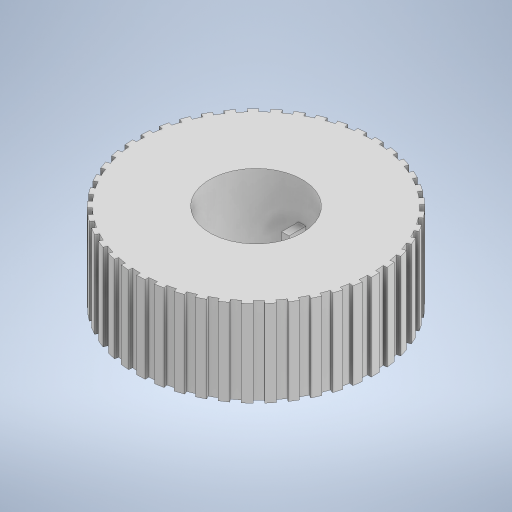
# Autodesk Inventor part: DialKnob
Saved by Autodesk Inventor 2024 (Build 280153000, 153)
## iProperties
Created: 2023-11-18
Part Number: DialKnob
Material: Generic
Document SubType Name: Modeling
Designer: gcter
Density: 1 g/cm^3
Appearance: Default
Author: gcter
Autodesk Inventor part; units mm, degrees
ref_plane "YZ Plane" through (0, 0, 0) normal (1, 0, 0) x (0, 1, 0)
ref_plane "XZ Plane" through (0, 0, 0) normal (0, 1, 0) x (-1, 0, 0)
ref_plane "XY Plane" through (0, 0, 0) normal (0, 0, 1) x (1, 0, 0)
sketch "Sketch1" plane through (0, 0, 0) normal (0, 1, 0) x (-1, 0, 0)
  arc A0 (-1.1143, -7.923) -> (-0.5589, -7.9815) centre (0, 0) ccw
  line L0 (-0.0008, -8.0004) -> (-0.0009, -8.255)
  line L1 (-0.5589, -7.9815) -> (-0.5767, -8.2348)
  circle A1 centre (0, 0) radius 8.255 construction
  line L2 (-0.0009, -8.255) -> (-0.5767, -8.2348)
  line L3 (-1.1143, -7.923) -> (-1.1497, -8.1745) construction
  line L4 (1.1126, -7.9227) -> (1.148, -8.1748)
  line L5 (1.148, -8.1748) -> (0.575, -8.235)
  line L6 (0.5573, -7.9816) -> (0.575, -8.235)
  arc A2 (-0.0008, -8.001) -> (0.5573, -7.9816) centre (0, 0) ccw
  line L7 (2.2044, -7.6907) -> (2.2746, -7.9355)
  line L8 (2.2746, -7.9355) -> (1.7155, -8.0748)
  line L9 (1.6627, -7.8263) -> (1.7155, -8.0748)
  arc A3 (1.1127, -7.9232) -> (1.6627, -7.8263) centre (0, 0) ccw
  line L10 (3.2533, -7.3091) -> (3.3568, -7.5417)
  line L11 (3.3568, -7.5417) -> (2.8226, -7.7575)
  line L12 (2.7357, -7.5188) -> (2.8226, -7.7575)
  arc A4 (2.2046, -7.6913) -> (2.7357, -7.5188) centre (0, 0) ccw
  line L13 (4.2389, -6.7852) -> (4.3738, -7.0011)
  line L14 (4.3738, -7.0011) -> (3.8747, -7.2891)
  line L15 (3.7555, -7.0649) -> (3.8747, -7.2891)
  arc A5 (3.2535, -7.3096) -> (3.7555, -7.0649) centre (0, 0) ccw
  line L16 (5.1419, -6.1292) -> (5.3056, -6.3242)
  line L17 (5.3056, -6.3242) -> (4.8515, -6.6789)
  line L18 (4.7022, -6.4734) -> (4.8515, -6.6789)
  arc A6 (4.2392, -6.7857) -> (4.7022, -6.4734) centre (0, 0) ccw
  line L19 (5.9449, -5.3539) -> (6.1341, -5.5243)
  line L20 (6.1341, -5.5243) -> (5.7338, -5.9387)
  line L21 (5.5574, -5.756) -> (5.7338, -5.9387)
  arc A7 (5.1423, -6.1297) -> (5.5574, -5.756) centre (0, 0) ccw
  line L22 (6.6322, -4.4745) -> (6.8432, -4.6168)
  line L23 (6.8432, -4.6168) -> (6.5045, -5.083)
  line L24 (6.3044, -4.9266) -> (6.5045, -5.083)
  arc A8 (5.9453, -5.3543) -> (6.3044, -4.9266) centre (0, 0) ccw
  line L25 (7.1904, -3.5079) -> (7.4192, -3.6195)
  line L26 (7.4192, -3.6195) -> (7.1486, -4.1282)
  line L27 (6.9287, -4.0012) -> (7.1486, -4.1282)
  arc A9 (6.6327, -4.4748) -> (6.9287, -4.0012) centre (0, 0) ccw
  line L28 (7.6086, -2.4731) -> (7.8507, -2.5517)
  line L29 (7.8507, -2.5517) -> (7.6536, -3.0932)
  line L30 (7.4181, -2.998) -> (7.6536, -3.0932)
  arc A10 (7.1909, -3.5082) -> (7.4181, -2.998) centre (0, 0) ccw
  line L31 (7.8787, -1.3901) -> (8.1294, -1.4343)
  line L32 (8.1294, -1.4343) -> (8.0096, -1.9979)
  line L33 (7.7631, -1.9364) -> (8.0096, -1.9979)
  arc A11 (7.6091, -2.4732) -> (7.7631, -1.9364) centre (0, 0) ccw
  line L34 (7.9955, -0.28) -> (8.2499, -0.2889)
  line L35 (8.2499, -0.2889) -> (8.2097, -0.8637)
  line L36 (7.9571, -0.8372) -> (8.2097, -0.8637)
  arc A12 (7.8793, -1.3902) -> (7.9571, -0.8372) centre (0, 0) ccw
  line L37 (7.9567, 0.8354) -> (8.2099, 0.862)
  line L38 (8.2099, 0.862) -> (8.25, 0.2872)
  line L39 (7.9962, 0.2784) -> (8.25, 0.2872)
  arc A13 (7.9961, -0.2801) -> (7.9962, 0.2784) centre (0, 0) ccw
  line L40 (7.763, 1.9347) -> (8.01, 1.9962)
  line L41 (8.01, 1.9962) -> (8.1297, 1.4326)
  line L42 (7.8796, 1.3885) -> (8.1297, 1.4326)
  arc A14 (7.9573, 0.8355) -> (7.8796, 1.3885) centre (0, 0) ccw
  line L43 (7.4182, 2.9962) -> (7.6542, 3.0916)
  line L44 (7.6542, 3.0916) -> (7.8512, 2.5501)
  line L45 (7.6097, 2.4717) -> (7.8512, 2.5501)
  arc A15 (7.7635, 1.9348) -> (7.6097, 2.4717) centre (0, 0) ccw
  line L46 (6.929, 3.9995) -> (7.1495, 4.1268)
  line L47 (7.1495, 4.1268) -> (7.4199, 3.618)
  line L48 (7.1916, 3.5067) -> (7.4199, 3.618)
  arc A16 (7.4187, 2.9965) -> (7.1916, 3.5067) centre (0, 0) ccw
  line L49 (6.3049, 4.9249) -> (6.5056, 5.0816)
  line L50 (6.5056, 5.0816) -> (6.8442, 4.6154)
  line L51 (6.6336, 4.4734) -> (6.8442, 4.6154)
  arc A17 (6.9295, 3.9998) -> (6.6336, 4.4734) centre (0, 0) ccw
  line L52 (5.5582, 5.7545) -> (5.735, 5.9376)
  line L53 (5.735, 5.9376) -> (6.1352, 5.523)
  line L54 (5.9465, 5.3531) -> (6.1352, 5.523)
  arc A18 (6.3054, 4.9253) -> (5.9465, 5.3531) centre (0, 0) ccw
  line L55 (4.7032, 6.472) -> (4.8529, 6.6779)
  line L56 (4.8529, 6.6779) -> (5.3069, 6.3231)
  line L57 (5.1436, 6.1286) -> (5.3069, 6.3231)
  arc A19 (5.5586, 5.7549) -> (5.1436, 6.1286) centre (0, 0) ccw
  line L58 (3.7567, 7.0636) -> (3.8762, 7.2883)
  line L59 (3.8762, 7.2883) -> (4.3752, 7.0002)
  line L60 (4.2406, 6.7848) -> (4.3752, 7.0002)
  arc A20 (4.7035, 6.4725) -> (4.2406, 6.7848) centre (0, 0) ccw
  line L61 (2.7371, 7.5177) -> (2.8242, 7.7569)
  line L62 (2.8242, 7.7569) -> (3.3584, 7.541)
  line L63 (3.2551, 7.3089) -> (3.3584, 7.541)
  arc A21 (3.757, 7.0641) -> (3.2551, 7.3089) centre (0, 0) ccw
  line L64 (1.6642, 7.8254) -> (1.7171, 8.0744)
  line L65 (1.7171, 8.0744) -> (2.2762, 7.935)
  line L66 (2.2062, 7.6908) -> (2.2762, 7.935)
  arc A22 (2.7373, 7.5182) -> (2.2062, 7.6908) centre (0, 0) ccw
  line L67 (0.5589, 7.9809) -> (0.5767, 8.2348)
  line L68 (0.5767, 8.2348) -> (1.1497, 8.1745)
  line L69 (1.1143, 7.923) -> (1.1497, 8.1745)
  arc A23 (1.6643, 7.826) -> (1.1143, 7.923) centre (0, 0) ccw
  line L70 (-0.5573, 7.981) -> (-0.575, 8.235)
  line L71 (-0.575, 8.235) -> (0.0009, 8.255)
  line L72 (0.0008, 8.001) -> (0.0009, 8.255)
  arc A24 (0.5589, 7.9815) -> (0.0008, 8.001) centre (0, 0) ccw
  line L73 (-1.6626, 7.8258) -> (-1.7155, 8.0748)
  line L74 (-1.7155, 8.0748) -> (-1.148, 8.1748)
  line L75 (-1.1127, 7.9232) -> (-1.148, 8.1748)
  arc A25 (-0.5573, 7.9816) -> (-1.1127, 7.9232) centre (0, 0) ccw
  line L76 (-2.7355, 7.5182) -> (-2.8226, 7.7575)
  line L77 (-2.8226, 7.7575) -> (-2.2746, 7.9355)
  line L78 (-2.2046, 7.6913) -> (-2.2746, 7.9355)
  arc A26 (-1.6627, 7.8263) -> (-2.2046, 7.6913) centre (0, 0) ccw
  line L79 (-3.7552, 7.0643) -> (-3.8747, 7.2891)
  line L80 (-3.8747, 7.2891) -> (-3.3568, 7.5417)
  line L81 (-3.2535, 7.3096) -> (-3.3568, 7.5417)
  arc A27 (-2.7357, 7.5188) -> (-3.2535, 7.3096) centre (0, 0) ccw
  line L82 (-4.7019, 6.473) -> (-4.8515, 6.6789)
  line L83 (-4.8515, 6.6789) -> (-4.3738, 7.0011)
  line L84 (-4.2392, 6.7857) -> (-4.3738, 7.0011)
  arc A28 (-3.7555, 7.0649) -> (-4.2392, 6.7857) centre (0, 0) ccw
  line L85 (-5.557, 5.7556) -> (-5.7338, 5.9387)
  line L86 (-5.7338, 5.9387) -> (-5.3056, 6.3242)
  line L87 (-5.1423, 6.1297) -> (-5.3056, 6.3242)
  arc A29 (-4.7022, 6.4734) -> (-5.1423, 6.1297) centre (0, 0) ccw
  line L88 (-6.3039, 4.9262) -> (-6.5045, 5.083)
  line L89 (-6.5045, 5.083) -> (-6.1341, 5.5243)
  line L90 (-5.9453, 5.3543) -> (-6.1341, 5.5243)
  arc A30 (-5.5574, 5.756) -> (-5.9453, 5.3543) centre (0, 0) ccw
  line L91 (-6.9282, 4.0009) -> (-7.1486, 4.1282)
  line L92 (-7.1486, 4.1282) -> (-6.8432, 4.6168)
  line L93 (-6.6327, 4.4748) -> (-6.8432, 4.6168)
  arc A31 (-6.3044, 4.9266) -> (-6.6327, 4.4748) centre (0, 0) ccw
  line L94 (-7.4176, 2.9978) -> (-7.6536, 3.0932)
  line L95 (-7.6536, 3.0932) -> (-7.4192, 3.6195)
  line L96 (-7.1909, 3.5082) -> (-7.4192, 3.6195)
  arc A32 (-6.9287, 4.0012) -> (-7.1909, 3.5082) centre (0, 0) ccw
  line L97 (-7.7626, 1.9363) -> (-8.0096, 1.9979)
  line L98 (-8.0096, 1.9979) -> (-7.8507, 2.5517)
  line L99 (-7.6091, 2.4732) -> (-7.8507, 2.5517)
  arc A33 (-7.4181, 2.998) -> (-7.6091, 2.4732) centre (0, 0) ccw
  line L100 (-7.9565, 0.8371) -> (-8.2097, 0.8637)
  line L101 (-8.2097, 0.8637) -> (-8.1294, 1.4343)
  line L102 (-7.8793, 1.3902) -> (-8.1294, 1.4343)
  arc A34 (-7.7631, 1.9364) -> (-7.8793, 1.3902) centre (0, 0) ccw
  line L103 (-7.9956, -0.2784) -> (-8.25, -0.2872)
  line L104 (-8.25, -0.2872) -> (-8.2499, 0.2889)
  line L105 (-7.9961, 0.2801) -> (-8.2499, 0.2889)
  arc A35 (-7.9571, 0.8372) -> (-7.9961, 0.2801) centre (0, 0) ccw
  line L106 (-7.879, -1.3884) -> (-8.1297, -1.4326)
  line L107 (-8.1297, -1.4326) -> (-8.2099, -0.862)
  line L108 (-7.9573, -0.8355) -> (-8.2099, -0.862)
  arc A36 (-7.9962, -0.2784) -> (-7.9573, -0.8355) centre (0, 0) ccw
  line L109 (-7.6091, -2.4715) -> (-7.8512, -2.5501)
  line L110 (-7.8512, -2.5501) -> (-8.01, -1.9962)
  line L111 (-7.7635, -1.9348) -> (-8.01, -1.9962)
  arc A37 (-7.8796, -1.3885) -> (-7.7635, -1.9348) centre (0, 0) ccw
  line L112 (-7.1911, -3.5064) -> (-7.4199, -3.618)
  line L113 (-7.4199, -3.618) -> (-7.6542, -3.0916)
  line L114 (-7.4187, -2.9965) -> (-7.6542, -3.0916)
  arc A38 (-7.6097, -2.4717) -> (-7.4187, -2.9965) centre (0, 0) ccw
  line L115 (-6.6331, -4.4731) -> (-6.8442, -4.6154)
  line L116 (-6.8442, -4.6154) -> (-7.1495, -4.1268)
  line L117 (-6.9295, -3.9998) -> (-7.1495, -4.1268)
  arc A39 (-7.1916, -3.5067) -> (-6.9295, -3.9998) centre (0, 0) ccw
  line L118 (-5.946, -5.3527) -> (-6.1352, -5.523)
  line L119 (-6.1352, -5.523) -> (-6.5056, -5.0816)
  line L120 (-6.3054, -4.9253) -> (-6.5056, -5.0816)
  arc A40 (-6.6336, -4.4734) -> (-6.3054, -4.9253) centre (0, 0) ccw
  line L121 (-5.1432, -6.1282) -> (-5.3069, -6.3231)
  line L122 (-5.3069, -6.3231) -> (-5.735, -5.9376)
  line L123 (-5.5586, -5.7549) -> (-5.735, -5.9376)
  arc A41 (-5.9465, -5.3531) -> (-5.5586, -5.7549) centre (0, 0) ccw
  line L124 (-4.2403, -6.7843) -> (-4.3752, -7.0002)
  line L125 (-4.3752, -7.0002) -> (-4.8529, -6.6779)
  line L126 (-4.7035, -6.4725) -> (-4.8529, -6.6779)
  arc A42 (-5.1436, -6.1286) -> (-4.7035, -6.4725) centre (0, 0) ccw
  line L127 (-3.2548, -7.3084) -> (-3.3584, -7.541)
  line L128 (-3.3584, -7.541) -> (-3.8762, -7.2883)
  line L129 (-3.757, -7.0641) -> (-3.8762, -7.2883)
  arc A43 (-4.2406, -6.7848) -> (-3.757, -7.0641) centre (0, 0) ccw
  line L130 (-2.206, -7.6903) -> (-2.2762, -7.935)
  line L131 (-2.2762, -7.935) -> (-2.8242, -7.7569)
  line L132 (-2.7373, -7.5182) -> (-2.8242, -7.7569)
  arc A44 (-3.2551, -7.3089) -> (-2.7373, -7.5182) centre (0, 0) ccw
  line L133 (-1.1143, -7.9225) -> (-1.1497, -8.1745)
  line L134 (-1.1497, -8.1745) -> (-1.7171, -8.0744)
  line L135 (-1.6643, -7.826) -> (-1.7171, -8.0744)
  arc A45 (-2.2062, -7.6908) -> (-1.6643, -7.826) centre (0, 0) ccw
  point P0 (-0.0008, -8.001)
  point P1 (1.1127, -7.9232)
  point P2 (2.2046, -7.6913)
  point P3 (3.2535, -7.3096)
  point P4 (4.2392, -6.7857)
  point P5 (5.1423, -6.1297)
  point P6 (5.9453, -5.3543)
  point P7 (6.6327, -4.4748)
  point P8 (7.1909, -3.5082)
  point P9 (7.6091, -2.4732)
  point P10 (7.8793, -1.3902)
  point P11 (7.9961, -0.2801)
  point P12 (7.9573, 0.8355)
  point P13 (7.7635, 1.9348)
  point P14 (7.4187, 2.9965)
  point P15 (6.9295, 3.9998)
  point P16 (6.3054, 4.9253)
  point P17 (5.5586, 5.7549)
  point P18 (4.7035, 6.4725)
  point P19 (3.757, 7.0641)
  point P20 (2.7373, 7.5182)
  point P21 (1.6643, 7.826)
  point P22 (0.5589, 7.9815)
  point P23 (-0.5573, 7.9816)
  point P24 (-1.6627, 7.8263)
  point P25 (-2.7357, 7.5188)
  point P26 (-3.7555, 7.0649)
  point P27 (-4.7022, 6.4734)
  point P28 (-5.5574, 5.756)
  point P29 (-6.3044, 4.9266)
  point P30 (-6.9287, 4.0012)
  point P31 (-7.4181, 2.998)
  point P32 (-7.7631, 1.9364)
  point P33 (-7.9571, 0.8372)
  point P34 (-7.9962, -0.2784)
  point P35 (-7.8796, -1.3885)
  point P36 (-7.6097, -2.4717)
  point P37 (-7.1916, -3.5067)
  point P38 (-6.6336, -4.4734)
  point P39 (-5.9465, -5.3531)
  point P40 (-5.1436, -6.1286)
  point P41 (-4.2406, -6.7848)
  point P42 (-3.2551, -7.3089)
  point P43 (-2.2062, -7.6908)
  point P44 (-1.1143, -7.923)
  dimension "d0" = 16.002
  dimension "d1" = 4
  dimension "d2" = 0.254
  dimension "d3" = 4
  dimension "d6" = 360
  constraints: 272 end point, 93 point on circle, 46 centre point, 3 line through centre, 2 coincident, 451 other
  measures "d0" diameter of A0
  measures "d1" angle of L1 L0
  measures "d2" radial gap between concentric circles of A0 A1
  measures "d3" angle of L1 L3
extrude "Extrusion1" add sketch "Sketch1" along normal blind 5.969
sketch "Sketch2" plane through (0, 5.969, 0) normal (0, 1, 0) x (1, 0, 0)
  arc A0 (-0.254, 3.1903) -> (0.254, 3.1903) centre (0, 0) ccw
  line L0 (0, 3.2004) -> (0, -3.2004) construction
  line L1 (-0.254, 2.032) -> (0.254, 2.032)
  line L2 (-0.254, 2.032) -> (-0.254, 3.1903)
  line L3 (0.254, 2.032) -> (0.254, 3.1903)
  dimension "d10" = 6.4008
  dimension "d13" = 0.254
  dimension "d14" = 0.254
  dimension "d16" = 2.032
  constraints: 8 end point, 3 point on circle, 2 coincident, 2 vertical, 1 centre point, 1 horizontal, 1 midpoint, 1 parallel
  measures "d10" diameter of A0
  measures "d13" distance from line of L1.end L0
  measures "d14" distance from line of L0 L1.start
  measures "d16" distance from line of point (0, 0) L1
extrude "Extrusion2" cut sketch "Sketch2" against normal blind 4.699
sketch "Sketch3" plane through (0, 5.969, 0) normal (0, 1, 0) x (1, 0, 0)
  circle A0 centre (0, 0) radius 3.2004
  arc A1 (-0.254, 3.1903) -> (0.254, 3.1903) centre (0, 0) ccw projected
  constraints: 1 centre point, 1 coincident, 1 concentric
extrude "Extrusion3" cut sketch "Sketch3" against normal blind 2.667
body "Solid1"
